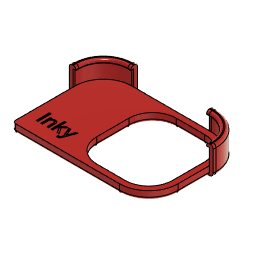
De-Anza-Merch-iPh-Case-Separate-Version v2 (Autodesk Fusion 360 design; units mm, degrees)
Autodesk Fusion 360 part; units mm, degrees
(part 1 of 2)
sketch "Body\\" plane through (0, 0, 0) normal (0, 0, 1) x (1, 0, 0)
  line L0 (0, 0) -> (72, 0)
  line L1 (0, 0) -> (0, 32)
  line L2 (0, 32) -> (-2, 32)
  line L3 (-2, 32) -> (-2, 33.5)
  line L4 (14.5, 50) -> (16, 50)
  line L5 (16, 50) -> (16, 48)
  line L6 (56, 48) -> (56, 50)
  line L7 (56, 50) -> (57.5, 50)
  line L8 (74, 33.5) -> (74, 32)
  line L9 (74, 32) -> (72, 32)
  line L10 (72, 32) -> (72, 0)
  line L11 (56.5, 3) -> (41.5, 3)
  line L12 (29, 15.5) -> (29, 32.5)
  line L13 (41.5, 45) -> (56.5, 45)
  line L14 (69, 32.5) -> (69, 15.5)
  line L15 (56, 48) -> (16, 48)
  arc A0 (14.5, 50) -> (-2, 33.5) centre (14.5, 33.5) ccw
  arc A1 (74, 33.5) -> (57.5, 50) centre (57.5, 33.5) ccw
  arc A2 (41.5, 45) -> (29, 32.5) centre (41.5, 32.5) ccw
  arc A3 (56.5, 3) -> (69, 15.5) centre (56.5, 15.5) ccw
  arc A4 (69, 32.5) -> (56.5, 45) centre (56.5, 32.5) ccw
  arc A5 (29, 15.5) -> (41.5, 3) centre (41.5, 15.5) ccw
  line L16 (32.6612, 41.3388) -> (65.3388, 6.6612) construction
  point P0 (74, 50)
  dimension "d2" = 72
  dimension "d3" = 40
  dimension "d5" = 42
  dimension "d6" = 3
  dimension "d15" = 48
  dimension "d16" = 3
  dimension "d27" = 16.5
  dimension "d28" = 16.5
  dimension "d29" = 12.5
  dimension "d30" = 12.5
  dimension "d31" = 2
  dimension "d32" = 2
  dimension "d33" = 2
  dimension "d34" = 2
  dimension "d35" = 12.5
  dimension "d36" = 12.5
  dimension "d38" = 18
  dimension "d39" = 18
  dimension "d40" = 18
  dimension "d41" = 18
  constraint perpendicular L1 L2
  constraint perpendicular L3 L4
  constraint perpendicular L4 L5
  constraint perpendicular L6 L7
  constraint perpendicular L7 L8
  constraint perpendicular L8 L9
  constraint perpendicular L0 L10
  constraint horizontal L11
  constraint vertical L12
  constraint horizontal L13
  constraint vertical L14
  constraint perpendicular L5 L15
  constraint coincident L0.start L1
  constraint coincident L5.end L15.end
  constraint coincident L0.start L1.start
  constraint coincident L1.start L0
  constraint tangent L4 A0
  constraint tangent L3 A0
  constraint coincident P0 L7
  constraint coincident P0 L8
  constraint tangent L7 A1
  constraint tangent L8 A1
  constraint tangent L13 A2
  constraint tangent L12 A2
  constraint tangent L11 A3
  constraint tangent L14 A3
  constraint vertical L6
  constraint tangent L13 A4
  constraint tangent L14 A4
  constraint tangent L11 A5
  constraint tangent L12 A5
  constraint midpoint A2 L16.start
  constraint midpoint A3 L16.end
  measures "d2" distance of L1 L10
  measures "d3" distance of L12 L14
  measures "d5" distance of L11 L13
  measures "d6" distance of L10 L14
  measures "d15" distance of L0 L15
  measures "d16" distance of L13 L15
  measures "d27" radius of A0
  measures "d28" radius of A1
  measures "d29" radius of A2
  measures "d30" radius of A3
  measures "d31" distance of L4 L15
  measures "d32" distance of L1 L3
  measures "d33" distance of L8 L10
  measures "d34" distance of L7 L15
  measures "d35" radius of A4
  measures "d36" radius of A5
  measures "d38" distance of L6 L8
  measures "d39" distance of L7 L9
  measures "d40" distance of L2 L4
  measures "d41" distance of L3 L5
extrude "Extrude1" add sketch "Body\\" along normal blind 4.5
sketch "Sketch5" plane through (0, 0, 4.5) normal (0, 0, 1) x (-1, 0, 0)
  arc A0 (-41.5, -45) -> (-29, -32.5) centre (-41.5, -32.5) ccw
  line L0 (-41.5, -45) -> (-56.5, -45)
  arc A1 (-69, -32.5) -> (-56.5, -45) centre (-56.5, -32.5) ccw
  line L1 (-69, -32.5) -> (-69, -15.5)
  arc A2 (-56.5, -3) -> (-69, -15.5) centre (-56.5, -15.5) ccw
  line L2 (-56.5, -3) -> (-41.5, -3)
  arc A3 (-29, -15.5) -> (-41.5, -3) centre (-41.5, -15.5) ccw
  line L3 (-29, -15.5) -> (-29, -32.5)
  line L4 (-74, -32) -> (-74, -33.5)
  arc A4 (-74, -33.5) -> (-57.5, -50) centre (-57.5, -33.5) ccw
  line L5 (-57.5, -50) -> (-56, -50)
  line L6 (-56, -50) -> (-56, -48)
  line L7 (-56, -48) -> (-16, -48)
  line L8 (-16, -48) -> (-16, -50)
  line L9 (-16, -50) -> (-14.5, -50)
  arc A5 (-14.5, -50) -> (2, -33.5) centre (-14.5, -33.5) ccw
  line L10 (2, -33.5) -> (2, -32)
  line L11 (2, -32) -> (0, -32)
  line L12 (0, -32) -> (0, 0)
  line L13 (0, 0) -> (-72, 0)
  line L14 (-72, 0) -> (-72, -32)
  line L15 (-72, -32) -> (-74, -32)
  line L16 (2, -32) -> (2, -33.5)
  line L17 (-14.5, -50) -> (-16, -50)
  line L18 (-16, -50) -> (-16, -46.5)
  line L19 (-1.5, -32) -> (-1.5, -33.5)
  line L20 (-14.5, -46.5) -> (-16, -46.5)
  line L21 (-1.5, -32) -> (2, -32)
  arc A6 (-14.5, -50) -> (2, -33.5) centre (-14.5, -33.5) ccw
  arc A7 (-14.5, -46.5) -> (-1.5, -33.5) centre (-14.5, -33.5) ccw
  line L22 (-36, -60) -> (-36, 25) construction
  line L23 (-56, -50) -> (-56, -46.5)
  arc A8 (-70.5, -33.5) -> (-57.5, -46.5) centre (-57.5, -33.5) ccw
  arc A9 (-74, -33.5) -> (-57.5, -50) centre (-57.5, -33.5) ccw
  line L24 (-57.5, -50) -> (-56, -50)
  line L25 (-57.5, -46.5) -> (-56, -46.5)
  line L26 (-70.5, -32) -> (-74, -32)
  line L27 (-74, -32) -> (-74, -33.5)
  line L28 (-70.5, -32) -> (-70.5, -33.5)
  dimension "d63" = 18
  dimension "d64" = 50
  dimension "d65" = 2
  dimension "d66" = 3.5
  dimension "d67" = 3.5
  dimension "d68" = 16.5
  dimension "d69" = 13
  dimension "d70" = 36
  constraint vertical L16
  constraint horizontal L17
  constraint vertical L18
  constraint vertical L19
  constraint horizontal L20
  constraint coincident L10.end L11.start
  constraint perpendicular L16 L21
  constraint tangent L16 A6
  constraint tangent L17 A6
  constraint tangent L19 A7
  constraint tangent L20 A7
  constraint vertical L22
  constraint symmetric L10.end L22 L4.start
  constraint symmetric L8.end L22 L5.end
  constraint symmetric L19.start L22 L26.start
  constraint symmetric L18.end L22 L23.end
  constraint symmetric A5.end L22 L4.end
  constraint symmetric L9.end L22 A4.end
  constraint symmetric A6 L22 A9
  constraint symmetric L19.end L22 A8.start
  constraint symmetric L20.start L22 A8.end
  constraint symmetric A7 L22 A8
  measures "d63" distance of L16 L18
  measures "d64" distance of L12.end L17
  measures "d65" distance of L12.end L16
  measures "d66" distance of L17 L20
  measures "d67" distance of L16 L19
  measures "d68" radius of A6
  measures "d69" radius of A7
  measures "d70" distance of L12.end L22
extrude "Extrude4" add sketch "Sketch5" along normal blind 10 contours L4 A4 L5 L6 L15 L23 A8 A9 L24 L25 L26 L27 L28 | L8 L9 A5 L10 L11 L16 L17 L18 L19 L20 L21 A6 A7
sketch "Sketch7" plane through (0, 0, 4.5) normal (0, 0, 1) x (-1, 0, 0)
  line L0 (-1.5, -32) -> (0, -32)
  line L1 (0, -32) -> (0, 0)
  line L2 (0, 0) -> (-72, 0)
  line L3 (-72, 0) -> (-72, -32)
  line L4 (-72, -32) -> (-70.5, -32)
  line L5 (-70.5, -32) -> (-70.5, -33.5)
  arc A0 (-70.5, -33.5) -> (-57.5, -46.5) centre (-57.5, -33.5) ccw
  line L6 (-57.5, -46.5) -> (-56, -46.5)
  line L7 (-56, -46.5) -> (-56, -48)
  line L8 (-56, -48) -> (-16, -48)
  line L9 (-16, -48) -> (-16, -46.5)
  line L10 (-16, -46.5) -> (-14.5, -46.5)
  arc A1 (-14.5, -46.5) -> (-1.5, -33.5) centre (-14.5, -33.5) ccw
  line L11 (-1.5, -33.5) -> (-1.5, -32)
  arc A2 (-41.5, -45) -> (-29, -32.5) centre (-41.5, -32.5) ccw
  line L12 (-41.5, -45) -> (-56.5, -45)
  arc A3 (-69, -32.5) -> (-56.5, -45) centre (-56.5, -32.5) ccw
  line L13 (-69, -32.5) -> (-69, -15.5)
  arc A4 (-56.5, -3) -> (-69, -15.5) centre (-56.5, -15.5) ccw
  line L14 (-56.5, -3) -> (-41.5, -3)
  arc A5 (-29, -15.5) -> (-41.5, -3) centre (-41.5, -15.5) ccw
  line L15 (-29, -15.5) -> (-29, -32.5)
  line L16 (0, -32) -> (-1.5, -32)
  line L17 (-16, -46.5) -> (-16, -48)
  line L18 (-16, -48) -> (-15, -48)
  line L19 (0, -33) -> (0, -32)
  line L20 (-1.5, -32) -> (-1.5, -33.5)
  line L21 (-14.5, -46.5) -> (-16, -46.5)
  arc A6 (-14.5, -46.5) -> (-1.5, -33.5) centre (-14.5, -33.5) ccw
  arc A7 (-15, -48) -> (0, -33) centre (-15, -33) ccw
  line L22 (-36, -60) -> (-36, 0) construction
  arc A8 (-70.5, -33.5) -> (-57.5, -46.5) centre (-57.5, -33.5) ccw
  line L23 (-70.5, -32) -> (-70.5, -33.5)
  arc A9 (-70.5, -33.5) -> (-57.5, -46.5) centre (-57.5, -33.5) ccw
  line L24 (-56, -46.5) -> (-56, -48)
  line L25 (-70.5, -32) -> (-72, -32)
  line L26 (-56, -48) -> (-57, -48)
  arc A10 (-72, -33) -> (-57, -48) centre (-57, -33) ccw
  line L27 (-72, -33) -> (-72, -32)
  line L28 (-57.5, -46.5) -> (-56, -46.5)
  line L29 (-72, -32) -> (-70.5, -32)
  line L30 (-56, -46.5) -> (-57.5, -46.5)
  line L31 (-56, -48) -> (-56, -46.5)
  line L32 (-70.5, -33.5) -> (-70.5, -32)
  dimension "d73" = 14.5
  dimension "d74" = 14.5
  dimension "d75" = 13
  dimension "d76" = 15
  dimension "d77" = 60
  dimension "d78" = 36
  constraint horizontal L16
  constraint vertical L17
  constraint horizontal L18
  constraint vertical L19
  constraint coincident L8.end L9.start
  constraint coincident L0.end L1.start
  constraint vertical L20
  constraint horizontal L21
  constraint tangent L20 A6
  constraint tangent L21 A6
  constraint tangent L18 A7
  constraint tangent L19 A7
  constraint vertical L22
  constraint coincident L2 L22.end
  constraint symmetric L0.start L22 L4.end
  constraint symmetric L0.end L22 L3.end
  constraint symmetric L8.end L22 L7.end
  constraint symmetric L9.end L22 L6.end
  constraint symmetric L10.end L22 A0.end
  constraint symmetric A1.end L22 L5.end
  constraint symmetric A1 L22 A9
  constraint symmetric A6 L22 A8
  constraint symmetric L18.end L22 L26.end
  constraint symmetric L19.start L22 A10.start
  constraint symmetric A7 L22 A10
  measures "d73" distance of L16 L21
  measures "d74" distance of L17 L20
  measures "d75" radius of A6
  measures "d76" radius of A7
  measures "d77" distance of L22.start L22.end
  measures "d78" distance of L1.end L22
extrude "Extrude5" cut sketch "Sketch7" along normal blind 8.3 contours L0 L9 L10 A1 L11 L16 L17 L18 L19 L20 L21 A6 A7 | L4 L5 A0 L6 L7 A8 L23 A9 L24 L25 L26 A10 L27 L28 L29 L30 L31 L32
fillet "Fillet1" radius 15.5 1 edges at (72, 0, 2.25)
fillet "Fillet2" radius 2 6 edges at (74, 32.75, 0) (69.1673, 45.1673, 0) (56.75, 50, 0) (15.25, 50, 0) (2.8327, 45.1673, 0) (-2, 32.75, 0)
fillet "Fillet3" radius 1.5 6 edges at (1.5, 32.75, 14.5) (5.3076, 42.6924, 14.5) (15.25, 46.5, 14.5) (56.75, 46.5, 14.5) (66.6924, 42.6924, 14.5) (70.5, 32.75, 14.5)
fillet "Fillet4" radius 1.5 6 edges at (15.25, 50, 14.5) (2.8327, 45.1673, 14.5) (-2, 32.75, 14.5) (74, 32.75, 14.5) (69.1673, 45.1673, 14.5) (56.75, 50, 14.5)
fillet "Fillet5" radius 1.5 8 edges at (69, 24, 0) (65.3388, 6.6612, 0) (49, 3, 0) (32.6612, 6.6612, 0) (29, 24, 0) (32.6612, 41.3388, 0) (49, 45, 0) (65.3388, 41.3388, 0)
fillet "Fillet6" radius 1.5 3 edges at (28.25, 0, 0) (67.4602, 4.5398, 0) (72, 23.75, 0)
fillet "Fillet7" radius 1.5 3 edges at (0, 0, 3) (0, 0.4393, 0.4393) (0, 16.75, 0)
sketch "Sketch8" plane through (0, 0, 0) normal (0, 0, -1) x (1, 0, 0)
  line L0 (1.5, -1.5) -> (1.5, -32)
  line L1 (1.5, -32) -> (0, -32)
  line L2 (0, -32) -> (0, -33.5)
  arc A0 (0, -33.5) -> (14.5, -48) centre (14.5, -33.5) ccw
  line L3 (14.5, -48) -> (16, -48)
  line L4 (16, -48) -> (56, -48)
  line L5 (56, -48) -> (57.5, -48)
  arc A1 (57.5, -48) -> (72, -33.5) centre (57.5, -33.5) ccw
  line L6 (72, -33.5) -> (72, -32)
  line L7 (72, -32) -> (70.5, -32)
  line L8 (70.5, -32) -> (70.5, -32.5)
  arc A2 (56.5, -46.5) -> (70.5, -32.5) centre (56.5, -32.5) ccw
  line L9 (56.5, -46.5) -> (41.5, -46.5)
  arc A3 (27.5, -32.5) -> (41.5, -46.5) centre (41.5, -32.5) ccw
  line L10 (27.5, -32.5) -> (27.5, -15.5)
  arc A4 (41.5, -1.5) -> (27.5, -15.5) centre (41.5, -15.5) ccw
  line L11 (41.5, -1.5) -> (1.5, -1.5)
  arc A5 (24.5, -32.5) -> (29.9783, -45) centre (41.5, -32.5) ccw
  line L12 (24.5, -32.5) -> (24.5, -15.5)
  arc A6 (28.5385, -4.5) -> (24.5, -15.5) centre (41.5, -15.5) ccw
  line L13 (28.5385, -4.5) -> (4.5, -4.5)
  line L14 (4.5, -4.5) -> (4.5, -35)
  line L15 (4.5, -35) -> (3.0982, -35)
  arc A7 (3.0982, -35) -> (14.5, -45) centre (14.5, -33.5) ccw
  line L16 (14.5, -45) -> (16, -45)
  line L17 (16, -45) -> (29.9783, -45)
  dimension "d95" = -3
extrude "Extrude6" cut sketch "Sketch8" against normal blind 1 contours A5 L12 A6 L13 L14 L15 A7 L16 L17
sketch "Sketch9" plane through (0, 0, 1) normal (0, 0, -1) x (1, 0, 0)
  line L0 (28.5385, -4.5) -> (4.5, -4.5)
  line L1 (4.5, -4.5) -> (4.5, -35)
  line L2 (4.5, -35) -> (3.0982, -35)
  arc A0 (3.0982, -35) -> (14.5, -45) centre (14.5, -33.5) ccw
  line L3 (14.5, -45) -> (29.9783, -45)
  arc A1 (24.5, -32.5) -> (29.9783, -45) centre (41.5, -32.5) ccw
  line L4 (24.5, -32.5) -> (24.5, -15.5)
  arc A2 (28.5385, -4.5) -> (24.5, -15.5) centre (41.5, -15.5) ccw
  spline S0 degree 3 poles (21.3936, -39.5443) (21.4725, -39.4567) (21.6302, -39.1939) (21.7353, -38.9574) knots 0 0 0 0 1 1 1 1
  spline S1 degree 3 poles (21.7353, -38.9574) (21.9018, -38.5894) (21.9368, -38.3704) (21.9368, -37.5994) knots 0 0 0 0 1 1 1 1
  spline S2 degree 3 poles (21.9368, -37.5994) (21.9368, -36.7233) (21.9193, -36.6532) (21.6477, -36.1538) knots 0 0 0 0 1 1 1 1
  spline S3 degree 3 poles (21.6477, -36.1538) (21.49, -35.8559) (21.1395, -35.3302) (20.8767, -34.971) knots 0 0 0 0 1 1 1 1
  spline S4 degree 3 poles (20.8767, -34.971) (20.4474, -34.4015) (20.4036, -34.3052) (20.4825, -34.1212) knots 0 0 0 0 1 1 1 1
  spline S5 degree 3 poles (20.4825, -34.1212) (20.6139, -33.8321) (20.6051, -33.0961) (20.4474, -32.3076) knots 0 0 0 0 1 1 1 1
  spline S6 degree 3 poles (20.4474, -32.3076) (20.2459, -31.2125) (19.7903, -30.3802) (19.2647, -30.1086) knots 0 0 0 0 1 1 1 1
  spline S7 degree 3 poles (19.2647, -30.1086) (19.1157, -30.0297) (18.923, -29.8195) (18.8354, -29.6355) knots 0 0 0 0 1 1 1 1
  spline S8 degree 3 poles (18.8354, -29.6355) (18.739, -29.4515) (18.4499, -29.1098) (18.1958, -28.8732) knots 0 0 0 0 1 1 1 1
  spline S9 degree 3 poles (18.1958, -28.8732) (17.7753, -28.4965) (17.6876, -28.3476) (17.4336, -27.6116) knots 0 0 0 0 1 1 1 1
  spline S10 degree 3 poles (17.4336, -27.6116) (17.0831, -26.6216) (16.6451, -25.728) (16.3297, -25.3513) knots 0 0 0 0 1 1 1 1
  spline S11 degree 3 poles (16.3297, -25.3513) (15.9792, -24.9307) (15.62, -24.8519) (14.1394, -24.8519) knots 0 0 0 0 1 1 1 1
  spline S12 degree 3 poles (14.1394, -24.8519) (12.65, -24.8606) (12.3433, -24.9395) (11.9578, -25.4389) knots 0 0 0 0 1 1 1 1
  spline S13 degree 3 poles (11.9578, -25.4389) (11.6775, -25.8068) (11.2219, -26.8056) (10.8977, -27.7431) knots 0 0 0 0 1 1 1 1
  spline S14 degree 3 poles (10.8977, -27.7431) (10.6962, -28.3301) (10.5823, -28.5053) (10.2319, -28.8207) knots 0 0 0 0 1 1 1 1
  spline S15 degree 3 poles (10.2319, -28.8207) (9.9953, -29.0309) (9.6975, -29.3814) (9.5748, -29.5917) knots 0 0 0 0 1 1 1 1
  spline S16 degree 3 poles (9.5748, -29.5917) (9.4434, -29.8107) (9.2331, -30.0385) (9.0929, -30.1086) knots 0 0 0 0 1 1 1 1
  spline S17 degree 3 poles (9.0929, -30.1086) (8.576, -30.3802) (8.1204, -31.2212) (7.9189, -32.3076) knots 0 0 0 0 1 1 1 1
  spline S18 degree 3 poles (7.9189, -32.3076) (7.7612, -33.0961) (7.7525, -33.7007) (7.8839, -34.0686) knots 0 0 0 0 1 1 1 1
  spline S19 degree 3 poles (7.8839, -34.0686) (7.9627, -34.3139) (7.9365, -34.384) (7.4896, -34.9798) knots 0 0 0 0 1 1 1 1
  spline S20 degree 3 poles (7.4896, -34.9798) (6.7099, -36.0048) (6.4558, -36.5656) (6.4033, -37.2927) knots 0 0 0 0 1 1 1 1
  spline S21 degree 3 poles (6.4033, -37.2927) (6.3595, -38.0024) (6.5259, -38.7033) (6.8501, -39.1851) knots 0 0 0 0 1 1 1 1
  spline S22 degree 3 poles (6.8501, -39.1851) (7.0253, -39.4567) (7.0954, -39.483) (7.5159, -39.5093) knots 0 0 0 0 1 1 1 1
  spline S23 degree 3 poles (7.5159, -39.5093) (8.0854, -39.5443) (8.6987, -39.3516) (9.2857, -38.9486) knots 0 0 0 0 1 1 1 1
  spline S24 degree 3 poles (9.2857, -38.9486) (9.6098, -38.7383) (9.7675, -38.677) (9.8727, -38.7296) knots 0 0 0 0 1 1 1 1
  spline S25 degree 3 poles (9.8727, -38.7296) (9.9603, -38.7734) (10.337, -38.896) (10.7225, -39.0099) knots 0 0 0 0 1 1 1 1
  spline S26 degree 3 poles (10.7225, -39.0099) (11.6775, -39.2815) (13.4648, -39.3078) (13.8853, -39.0537) knots 0 0 0 0 1 1 1 1
  spline S27 degree 3 poles (13.8853, -39.0537) (14.1569, -38.896) (14.1744, -38.896) (14.5424, -39.045) knots 0 0 0 0 1 1 1 1
  spline S28 degree 3 poles (14.5424, -39.045) (15.3747, -39.3779) (16.8378, -39.2903) (18.2046, -38.8259) knots 0 0 0 0 1 1 1 1
  line L5 (18.2046, -38.8259) -> (18.6864, -38.6682)
  line L6 (18.6864, -38.6682) -> (18.9931, -38.9135)
  spline S29 degree 3 poles (18.9931, -38.9135) (19.8779, -39.6144) (21.0519, -39.9211) (21.3936, -39.5443) knots 0 0 0 0 1 1 1 1
  spline S30 degree 3 poles (20.1671, -38.8172) (19.9655, -38.7208) (19.5976, -38.458) (19.361, -38.2477) knots 0 0 0 0 1 1 1 1
  spline S31 degree 3 poles (19.361, -38.2477) (18.9405, -37.8622) (18.9142, -37.8534) (18.6777, -37.9761) knots 0 0 0 0 1 1 1 1
  spline S32 degree 3 poles (18.6777, -37.9761) (18.5462, -38.0462) (18.0731, -38.2302) (17.6438, -38.3879) knots 0 0 0 0 1 1 1 1
  spline S33 degree 3 poles (17.6438, -38.3879) (16.9692, -38.6332) (16.6976, -38.677) (15.7865, -38.712) knots 0 0 0 0 1 1 1 1
  spline S34 degree 3 poles (15.7865, -38.712) (14.7527, -38.7646) (14.7176, -38.7558) (14.5073, -38.5456) knots 0 0 0 0 1 1 1 1
  spline S35 degree 3 poles (14.5073, -38.5456) (14.3934, -38.4317) (14.2708, -38.274) (14.2357, -38.2039) knots 0 0 0 0 1 1 1 1
  spline S36 degree 3 poles (14.2357, -38.2039) (14.1919, -38.0988) (14.1744, -38.0988) (14.1306, -38.2039) knots 0 0 0 0 1 1 1 1
  spline S37 degree 3 poles (14.1306, -38.2039) (14.0956, -38.274) (13.9729, -38.4317) (13.859, -38.5456) knots 0 0 0 0 1 1 1 1
  spline S38 degree 3 poles (13.859, -38.5456) (13.6487, -38.7558) (13.6137, -38.7558) (12.6237, -38.7208) knots 0 0 0 0 1 1 1 1
  spline S39 degree 3 poles (12.6237, -38.7208) (11.7651, -38.6858) (11.4585, -38.6332) (10.7576, -38.3966) knots 0 0 0 0 1 1 1 1
  spline S40 degree 3 poles (10.7576, -38.3966) (10.2932, -38.2389) (9.8026, -38.0374) (9.6624, -37.9586) knots 0 0 0 0 1 1 1 1
  line L7 (9.6624, -37.9586) -> (9.4083, -37.8009)
  line L8 (9.4083, -37.8009) -> (8.8827, -38.2915)
  spline S41 degree 3 poles (8.8827, -38.2915) (8.3044, -38.8259) (7.7087, -39.0975) (7.4546, -38.9486) knots 0 0 0 0 1 1 1 1
  spline S42 degree 3 poles (7.4546, -38.9486) (7.148, -38.7646) (6.9114, -38.125) (6.9114, -37.4592) knots 0 0 0 0 1 1 1 1
  spline S43 degree 3 poles (6.9114, -37.4592) (6.9114, -36.8897) (6.9377, -36.7933) (7.2443, -36.3202) knots 0 0 0 0 1 1 1 1
  spline S44 degree 3 poles (7.2443, -36.3202) (7.4371, -36.0311) (7.8226, -35.523) (8.1117, -35.19) knots 0 0 0 0 1 1 1 1
  spline S45 degree 3 poles (8.1117, -35.19) (8.7863, -34.3928) (8.7775, -34.4103) (8.6111, -34.0861) knots 0 0 0 0 1 1 1 1
  spline S46 degree 3 poles (8.6111, -34.0861) (8.4008, -33.6656) (8.4797, -32.5442) (8.7775, -31.8871) knots 0 0 0 0 1 1 1 1
  spline S47 degree 3 poles (8.7775, -31.8871) (8.9878, -31.414) (9.6449, -30.5904) (9.8114, -30.5904) knots 0 0 0 0 1 1 1 1
  spline S48 degree 3 poles (9.8114, -30.5904) (9.8552, -30.5904) (9.8902, -30.7394) (9.8902, -30.9234) knots 0 0 0 0 1 1 1 1
  spline S49 degree 3 poles (9.8902, -30.9234) (9.8902, -31.3264) (10.1443, -31.8783) (10.4422, -32.1587) knots 0 0 0 0 1 1 1 1
  spline S50 degree 3 poles (10.4422, -32.1587) (10.6524, -32.3514) (10.7225, -32.3602) (11.3095, -32.3164) knots 0 0 0 0 1 1 1 1
  spline S51 degree 3 poles (11.3095, -32.3164) (11.66, -32.2901) (12.0192, -32.2463) (12.098, -32.2113) knots 0 0 0 0 1 1 1 1
  spline S52 degree 3 poles (12.098, -32.2113) (12.2382, -32.1587) (12.2557, -32.2025) (12.2557, -32.5705) knots 0 0 0 0 1 1 1 1
  spline S53 degree 3 poles (12.2557, -32.5705) (12.2557, -32.807) (12.3346, -33.3152) (12.4222, -33.7007) knots 0 0 0 0 1 1 1 1
  spline S54 degree 3 poles (12.4222, -33.7007) (12.5186, -34.0861) (12.5799, -34.4103) (12.5624, -34.4278) knots 0 0 0 0 1 1 1 1
  spline S55 degree 3 poles (12.5624, -34.4278) (12.5448, -34.4453) (12.4572, -34.4191) (12.3609, -34.3665) knots 0 0 0 0 1 1 1 1
  spline S56 degree 3 poles (12.3609, -34.3665) (12.1068, -34.2351) (11.4672, -34.2526) (11.2044, -34.4015) knots 0 0 0 0 1 1 1 1
  spline S57 degree 3 poles (11.2044, -34.4015) (10.9415, -34.5505) (10.4772, -34.568) (10.2144, -34.4366) knots 0 0 0 0 1 1 1 1
  spline S58 degree 3 poles (10.2144, -34.4366) (10.0304, -34.3402) (10.0304, -34.349) (10.2319, -34.568) knots 0 0 0 0 1 1 1 1
  spline S59 degree 3 poles (10.2319, -34.568) (10.3545, -34.6907) (10.5035, -34.7958) (10.5736, -34.7958) knots 0 0 0 0 1 1 1 1
  spline S60 degree 3 poles (10.5736, -34.7958) (10.6612, -34.7958) (10.6787, -34.8484) (10.6349, -34.9535) knots 0 0 0 0 1 1 1 1
  spline S61 degree 3 poles (10.6349, -34.9535) (10.5999, -35.0323) (10.5122, -35.2777) (10.4509, -35.4879) knots 0 0 0 0 1 1 1 1
  spline S62 degree 3 poles (10.4509, -35.4879) (10.3808, -35.707) (10.2669, -35.9786) (10.1881, -36.0924) knots 0 0 0 0 1 1 1 1
  spline S63 degree 3 poles (10.1881, -36.0924) (9.9866, -36.3991) (10.0829, -36.4166) (10.5561, -36.1275) knots 0 0 0 0 1 1 1 1
  spline S64 degree 3 poles (10.5561, -36.1275) (10.8627, -35.9435) (11.143, -35.8559) (11.5198, -35.8209) knots 0 0 0 0 1 1 1 1
  spline S65 degree 3 poles (11.5198, -35.8209) (11.8089, -35.7946) (12.1769, -35.7157) (12.3258, -35.6369) knots 0 0 0 0 1 1 1 1
  line L9 (12.3258, -35.6369) -> (12.6062, -35.4879)
  line L10 (12.6062, -35.4879) -> (12.6149, -35.7332)
  spline S66 degree 3 poles (12.6149, -35.7332) (12.6149, -35.9698) (12.6237, -35.961) (12.7814, -35.6281) knots 0 0 0 0 1 1 1 1
  spline S67 degree 3 poles (12.7814, -35.6281) (12.9917, -35.1725) (12.9917, -34.6381) (12.7814, -33.8321) knots 0 0 0 0 1 1 1 1
  spline S68 degree 3 poles (12.7814, -33.8321) (12.5273, -32.8508) (12.501, -32.8946) (13.2808, -32.8333) knots 0 0 0 0 1 1 1 1
  spline S69 degree 3 poles (13.2808, -32.8333) (14.1306, -32.7632) (14.2357, -32.7632) (15.0768, -32.8333) knots 0 0 0 0 1 1 1 1
  spline S70 degree 3 poles (15.0768, -32.8333) (15.8741, -32.8946) (15.8478, -32.8508) (15.585, -33.8846) knots 0 0 0 0 1 1 1 1
  spline S71 degree 3 poles (15.585, -33.8846) (15.3747, -34.7345) (15.3659, -34.9973) (15.5587, -35.5493) knots 0 0 0 0 1 1 1 1
  spline S72 degree 3 poles (15.5587, -35.5493) (15.6989, -35.9347) (15.7164, -35.9523) (15.7427, -35.742) knots 0 0 0 0 1 1 1 1
  spline S73 degree 3 poles (15.7427, -35.742) (15.7602, -35.6018) (15.7777, -35.4967) (15.7952, -35.4967) knots 0 0 0 0 1 1 1 1
  spline S74 degree 3 poles (15.7952, -35.4967) (15.804, -35.4967) (15.9617, -35.5755) (16.1544, -35.6719) knots 0 0 0 0 1 1 1 1
  spline S75 degree 3 poles (16.1544, -35.6719) (16.3647, -35.777) (16.6713, -35.8471) (16.9605, -35.8471) knots 0 0 0 0 1 1 1 1
  spline S76 degree 3 poles (16.9605, -35.8471) (17.3284, -35.8471) (17.4949, -35.8997) (17.8191, -36.1187) knots 0 0 0 0 1 1 1 1
  spline S77 degree 3 poles (17.8191, -36.1187) (18.0381, -36.2677) (18.2396, -36.3728) (18.2659, -36.3465) knots 0 0 0 0 1 1 1 1
  spline S78 degree 3 poles (18.2659, -36.3465) (18.2834, -36.329) (18.2396, -36.1888) (18.152, -36.0311) knots 0 0 0 0 1 1 1 1
  spline S79 degree 3 poles (18.152, -36.0311) (18.0381, -35.8384) (17.933, -35.7595) (17.7665, -35.7595) knots 0 0 0 0 1 1 1 1
  spline S80 degree 3 poles (17.7665, -35.7595) (17.5124, -35.7595) (17.3372, -35.6106) (17.3372, -35.4003) knots 0 0 0 0 1 1 1 1
  spline S81 degree 3 poles (17.3372, -35.4003) (17.3372, -34.9447) (16.61, -34.5768) (16.1282, -34.787) knots 0 0 0 0 1 1 1 1
  line L11 (16.1282, -34.787) -> (15.8916, -34.8834)
  line L12 (15.8916, -34.8834) -> (16.1019, -34.7082)
  spline S82 degree 3 poles (16.1019, -34.7082) (16.2333, -34.5943) (16.4348, -34.533) (16.6538, -34.533) knots 0 0 0 0 1 1 1 1
  spline S83 degree 3 poles (16.6538, -34.533) (17.013, -34.533) (17.346, -34.7783) (17.7052, -35.3215) knots 0 0 0 0 1 1 1 1
  spline S84 degree 3 poles (17.7052, -35.3215) (17.8366, -35.523) (17.8541, -35.523) (17.8541, -35.3653) knots 0 0 0 0 1 1 1 1
  spline S85 degree 3 poles (17.8541, -35.3653) (17.8629, -35.2689) (17.8278, -35.1287) (17.7753, -35.0586) knots 0 0 0 0 1 1 1 1
  spline S86 degree 3 poles (17.7753, -35.0586) (17.7227, -34.9623) (17.7665, -34.8746) (17.9768, -34.6994) knots 0 0 0 0 1 1 1 1
  line L13 (17.9768, -34.6994) -> (18.2571, -34.4629)
  line L14 (18.2571, -34.4629) -> (17.8541, -34.5067)
  spline S87 degree 3 poles (17.8541, -34.5067) (17.5825, -34.5417) (17.3635, -34.5067) (17.1795, -34.4103) knots 0 0 0 0 1 1 1 1
  spline S88 degree 3 poles (17.1795, -34.4103) (16.8641, -34.2526) (16.2683, -34.2263) (16.0055, -34.3665) knots 0 0 0 0 1 1 1 1
  spline S89 degree 3 poles (16.0055, -34.3665) (15.9091, -34.4191) (15.8215, -34.4453) (15.804, -34.4278) knots 0 0 0 0 1 1 1 1
  spline S90 degree 3 poles (15.804, -34.4278) (15.7865, -34.4103) (15.8478, -34.0861) (15.9354, -33.7007) knots 0 0 0 0 1 1 1 1
  spline S91 degree 3 poles (15.9354, -33.7007) (16.0318, -33.3152) (16.1019, -32.807) (16.1106, -32.5705) knots 0 0 0 0 1 1 1 1
  spline S92 degree 3 poles (16.1106, -32.5705) (16.1106, -32.2025) (16.1282, -32.1587) (16.2596, -32.2113) knots 0 0 0 0 1 1 1 1
  spline S93 degree 3 poles (16.2596, -32.2113) (16.3472, -32.2463) (16.7064, -32.2989) (17.0568, -32.3251) knots 0 0 0 0 1 1 1 1
  spline S94 degree 3 poles (17.0568, -32.3251) (17.6701, -32.3602) (17.7052, -32.3602) (17.968, -32.1149) knots 0 0 0 0 1 1 1 1
  spline S95 degree 3 poles (17.968, -32.1149) (18.3009, -31.7995) (18.4761, -31.3965) (18.4761, -30.9409) knots 0 0 0 0 1 1 1 1
  spline S96 degree 3 poles (18.4761, -30.9409) (18.4761, -30.7481) (18.5112, -30.5904) (18.555, -30.5904) knots 0 0 0 0 1 1 1 1
  spline S97 degree 3 poles (18.555, -30.5904) (18.7127, -30.5904) (19.3785, -31.414) (19.5976, -31.8871) knots 0 0 0 0 1 1 1 1
  spline S98 degree 3 poles (19.5976, -31.8871) (19.8867, -32.5354) (19.9743, -33.6568) (19.7553, -34.0774) knots 0 0 0 0 1 1 1 1
  spline S99 degree 3 poles (19.7553, -34.0774) (19.6764, -34.2263) (19.6151, -34.3665) (19.6151, -34.3928) knots 0 0 0 0 1 1 1 1
  spline S100 degree 3 poles (19.6151, -34.3928) (19.6151, -34.4103) (19.9042, -34.7695) (20.2459, -35.1725) knots 0 0 0 0 1 1 1 1
  spline S101 degree 3 poles (20.2459, -35.1725) (21.1133, -36.1801) (21.5426, -36.916) (21.5426, -37.3979) knots 0 0 0 0 1 1 1 1
  spline S102 degree 3 poles (21.5426, -37.3979) (21.5426, -37.8622) (21.3148, -38.5456) (21.0782, -38.8084) knots 0 0 0 0 1 1 1 1
  spline S103 degree 3 poles (21.0782, -38.8084) (20.8592, -39.045) (20.6489, -39.0537) (20.1671, -38.8172) knots 0 0 0 0 1 1 1 1
  spline S104 degree 3 poles (10.7576, -35.2514) (11.0116, -34.752) (11.327, -34.533) (11.7739, -34.533) knots 0 0 0 0 1 1 1 1
  spline S105 degree 3 poles (11.7739, -34.533) (12.0367, -34.533) (12.1856, -34.5855) (12.3083, -34.7169) knots 0 0 0 0 1 1 1 1
  spline S106 degree 3 poles (12.3083, -34.7169) (12.4747, -34.9009) (12.4747, -34.9009) (12.2382, -34.7958) knots 0 0 0 0 1 1 1 1
  spline S107 degree 3 poles (12.2382, -34.7958) (11.7476, -34.568) (11.0292, -34.9447) (11.0292, -35.4266) knots 0 0 0 0 1 1 1 1
  spline S108 degree 3 poles (11.0292, -35.4266) (11.0292, -35.5931) (10.6612, -35.8033) (10.6086, -35.6719) knots 0 0 0 0 1 1 1 1
  spline S109 degree 3 poles (10.6086, -35.6719) (10.5911, -35.6281) (10.6612, -35.4441) (10.7576, -35.2514) knots 0 0 0 0 1 1 1 1
  spline S110 degree 3 poles (16.5837, -35.19) (16.5925, -34.8308) (16.6626, -34.8046) (16.8466, -35.0762) knots 0 0 0 0 1 1 1 1
  spline S111 degree 3 poles (16.8466, -35.0762) (17.0393, -35.3565) (17.0218, -35.4967) (16.7852, -35.4967) knots 0 0 0 0 1 1 1 1
  spline S112 degree 3 poles (16.7852, -35.4967) (16.61, -35.4967) (16.5837, -35.4529) (16.5837, -35.19) knots 0 0 0 0 1 1 1 1
  spline S113 degree 3 poles (11.3796, -35.3828) (11.3796, -35.2514) (11.6249, -34.8834) (11.7125, -34.8834) knots 0 0 0 0 1 1 1 1
  spline S114 degree 3 poles (11.7125, -34.8834) (11.7476, -34.8834) (11.7739, -35.0236) (11.7826, -35.19) knots 0 0 0 0 1 1 1 1
  spline S115 degree 3 poles (11.7826, -35.19) (11.7826, -35.4529) (11.7563, -35.4967) (11.5811, -35.4967) knots 0 0 0 0 1 1 1 1
  spline S116 degree 3 poles (11.5811, -35.4967) (11.4672, -35.4967) (11.3796, -35.4441) (11.3796, -35.3828) knots 0 0 0 0 1 1 1 1
  spline S117 degree 3 poles (16.0843, -31.8696) (15.7339, -31.7557) (15.2608, -31.6418) (15.033, -31.6067) knots 0 0 0 0 1 1 1 1
  spline S118 degree 3 poles (15.033, -31.6067) (14.3496, -31.5191) (14.2708, -31.449) (14.2708, -30.8971) knots 0 0 0 0 1 1 1 1
  spline S119 degree 3 poles (14.2708, -30.8971) (14.2708, -30.4327) (14.2795, -30.4152) (14.5073, -30.4152) knots 0 0 0 0 1 1 1 1
  spline S120 degree 3 poles (14.5073, -30.4152) (15.0505, -30.4152) (15.8303, -30.091) (16.5487, -29.5741) knots 0 0 0 0 1 1 1 1
  spline S121 degree 3 poles (16.5487, -29.5741) (17.0218, -29.2412) (17.1444, -29.2149) (17.5299, -29.4164) knots 0 0 0 0 1 1 1 1
  line L15 (17.5299, -29.4164) -> (17.8103, -29.5654)
  line L16 (17.8103, -29.5654) -> (17.2496, -29.8107)
  spline S122 degree 3 poles (17.2496, -29.8107) (16.9429, -29.9509) (16.7152, -30.091) (16.7502, -30.1173) knots 0 0 0 0 1 1 1 1
  spline S123 degree 3 poles (16.7502, -30.1173) (16.7765, -30.1436) (17.0043, -30.1173) (17.2671, -30.0648) knots 0 0 0 0 1 1 1 1
  spline S124 degree 3 poles (17.2671, -30.0648) (17.8716, -29.9246) (18.1607, -29.9684) (18.1958, -30.1962) knots 0 0 0 0 1 1 1 1
  spline S125 degree 3 poles (18.1958, -30.1962) (18.2133, -30.3539) (18.1432, -30.3889) (17.5387, -30.4853) knots 0 0 0 0 1 1 1 1
  spline S126 degree 3 poles (17.5387, -30.4853) (16.5662, -30.6342) (16.5224, -30.7657) (17.4511, -30.7657) knots 0 0 0 0 1 1 1 1
  line L17 (17.4511, -30.7657) -> (18.2133, -30.7657)
  line L18 (18.2133, -30.7657) -> (18.2133, -31.0197)
  spline S127 degree 3 poles (18.2133, -31.0197) (18.2133, -31.3176) (18.0293, -31.3789) (16.9955, -31.3877) knots 0 0 0 0 1 1 1 1
  spline S128 degree 3 poles (16.9955, -31.3877) (16.1106, -31.3965) (16.4348, -31.5366) (17.3547, -31.5454) knots 0 0 0 0 1 1 1 1
  spline S129 degree 3 poles (17.3547, -31.5454) (17.7314, -31.5542) (18.0381, -31.5804) (18.0381, -31.6155) knots 0 0 0 0 1 1 1 1
  spline S130 degree 3 poles (18.0381, -31.6155) (18.0381, -31.6505) (17.9505, -31.7644) (17.8453, -31.8783) knots 0 0 0 0 1 1 1 1
  spline S131 degree 3 poles (17.8453, -31.8783) (17.5913, -32.1499) (16.9254, -32.1499) (16.0843, -31.8696) knots 0 0 0 0 1 1 1 1
  spline S132 degree 3 poles (10.5298, -31.8871) (10.4159, -31.782) (10.3283, -31.6681) (10.3283, -31.6243) knots 0 0 0 0 1 1 1 1
  spline S133 degree 3 poles (10.3283, -31.6243) (10.3283, -31.5892) (10.6349, -31.5542) (11.0029, -31.5454) knots 0 0 0 0 1 1 1 1
  spline S134 degree 3 poles (11.0029, -31.5454) (11.9666, -31.5366) (12.2382, -31.3965) (11.3358, -31.3789) knots 0 0 0 0 1 1 1 1
  spline S135 degree 3 poles (11.3358, -31.3789) (10.3896, -31.3527) (10.2056, -31.3001) (10.1706, -31.0022) knots 0 0 0 0 1 1 1 1
  line L19 (10.1706, -31.0022) -> (10.1443, -30.7657)
  line L20 (10.1443, -30.7657) -> (10.9065, -30.7657)
  spline S136 degree 3 poles (10.9065, -30.7657) (11.8439, -30.7657) (11.8001, -30.643) (10.8276, -30.4853) knots 0 0 0 0 1 1 1 1
  spline S137 degree 3 poles (10.8276, -30.4853) (10.1706, -30.3889) (10.0742, -30.3188) (10.2319, -30.0735) knots 0 0 0 0 1 1 1 1
  spline S138 degree 3 poles (10.2319, -30.0735) (10.3283, -29.9246) (10.9503, -29.9772) (11.5811, -30.1962) knots 0 0 0 0 1 1 1 1
  spline S139 degree 3 poles (11.5811, -30.1962) (12.0192, -30.3451) (12.282, -30.3101) (11.8965, -30.1611) knots 0 0 0 0 1 1 1 1
  spline S140 degree 3 poles (11.8965, -30.1611) (11.7826, -30.1173) (11.4322, -29.9596) (11.1255, -29.8195) knots 0 0 0 0 1 1 1 1
  line L21 (11.1255, -29.8195) -> (10.5561, -29.5654)
  line L22 (10.5561, -29.5654) -> (10.8364, -29.4164)
  spline S141 degree 3 poles (10.8364, -29.4164) (11.2219, -29.2149) (11.3446, -29.2412) (11.8177, -29.5741) knots 0 0 0 0 1 1 1 1
  spline S142 degree 3 poles (11.8177, -29.5741) (12.5361, -30.091) (13.3158, -30.4152) (13.8503, -30.4152) knots 0 0 0 0 1 1 1 1
  spline S143 degree 3 poles (13.8503, -30.4152) (14.0868, -30.4152) (14.0956, -30.4327) (14.0956, -30.9058) knots 0 0 0 0 1 1 1 1
  spline S144 degree 3 poles (14.0956, -30.9058) (14.0956, -31.3702) (14.0868, -31.3877) (13.7889, -31.5191) knots 0 0 0 0 1 1 1 1
  spline S145 degree 3 poles (13.7889, -31.5191) (13.6225, -31.5804) (13.3596, -31.6418) (13.2019, -31.6418) knots 0 0 0 0 1 1 1 1
  spline S146 degree 3 poles (13.2019, -31.6418) (13.0442, -31.6505) (12.6324, -31.7469) (12.2995, -31.8608) knots 0 0 0 0 1 1 1 1
  spline S147 degree 3 poles (12.2995, -31.8608) (11.4935, -32.1412) (10.8101, -32.1499) (10.5298, -31.8871) knots 0 0 0 0 1 1 1 1
  line L23 (15.3221, -29.1273) -> (15.3309, -28.4439)
  line L24 (15.3309, -28.4439) -> (15.4973, -28.6455)
  spline S148 degree 3 poles (15.4973, -28.6455) (15.7602, -28.9609) (15.9004, -29.5041) (15.7602, -29.6705) knots 0 0 0 0 1 1 1 1
  spline S149 degree 3 poles (15.7602, -29.6705) (15.6989, -29.7406) (15.5762, -29.8019) (15.4886, -29.8019) knots 0 0 0 0 1 1 1 1
  spline S150 degree 3 poles (15.4886, -29.8019) (15.3396, -29.8019) (15.3221, -29.7318) (15.3221, -29.1273) knots 0 0 0 0 1 1 1 1
  spline S151 degree 3 poles (12.6062, -29.6705) (12.5098, -29.5566) (12.5186, -29.469) (12.6149, -29.1711) knots 0 0 0 0 1 1 1 1
  spline S152 degree 3 poles (12.6149, -29.1711) (12.6763, -28.9784) (12.7989, -28.7331) (12.8865, -28.6279) knots 0 0 0 0 1 1 1 1
  spline S153 degree 3 poles (12.8865, -28.6279) (13.0355, -28.4527) (13.0355, -28.4615) (13.0442, -29.1273) knots 0 0 0 0 1 1 1 1
  spline S154 degree 3 poles (13.0442, -29.1273) (13.0442, -29.7318) (13.0267, -29.8019) (12.8778, -29.8019) knots 0 0 0 0 1 1 1 1
  spline S155 degree 3 poles (12.8778, -29.8019) (12.7901, -29.8019) (12.6675, -29.7406) (12.6062, -29.6705) knots 0 0 0 0 1 1 1 1
  spline S156 degree 3 poles (16.829, -28.6455) (16.7852, -28.5841) (16.4786, -28.0234) (16.1544, -27.4101) knots 0 0 0 0 1 1 1 1
  line L25 (16.1544, -27.4101) -> (15.5587, -26.2799)
  line L26 (15.5587, -26.2799) -> (15.1995, -26.3413)
  spline S157 degree 3 poles (15.1995, -26.3413) (14.7176, -26.4201) (13.5962, -26.4201) (13.237, -26.3413) knots 0 0 0 0 1 1 1 1
  spline S158 degree 3 poles (13.237, -26.3413) (12.8515, -26.2537) (12.7726, -26.3413) (12.2557, -27.34) knots 0 0 0 0 1 1 1 1
  spline S159 degree 3 poles (12.2557, -27.34) (11.7038, -28.4177) (11.4935, -28.7506) (11.3796, -28.7506) knots 0 0 0 0 1 1 1 1
  spline S160 degree 3 poles (11.3796, -28.7506) (11.2394, -28.7506) (11.2745, -28.4702) (11.5198, -27.7343) knots 0 0 0 0 1 1 1 1
  spline S161 degree 3 poles (11.5198, -27.7343) (11.8702, -26.683) (12.2908, -25.8244) (12.5624, -25.6141) knots 0 0 0 0 1 1 1 1
  spline S162 degree 3 poles (12.5624, -25.6141) (12.7901, -25.4301) (12.8953, -25.4213) (14.1919, -25.4213) knots 0 0 0 0 1 1 1 1
  spline S163 degree 3 poles (14.1919, -25.4213) (15.5587, -25.4213) (15.5762, -25.4213) (15.8478, -25.6579) knots 0 0 0 0 1 1 1 1
  spline S164 degree 3 poles (15.8478, -25.6579) (15.9967, -25.7806) (16.2245, -26.1047) (16.3472, -26.3763) knots 0 0 0 0 1 1 1 1
  spline S165 degree 3 poles (16.3472, -26.3763) (16.6451, -27.0422) (17.0744, -28.3388) (17.0744, -28.5666) knots 0 0 0 0 1 1 1 1
  spline S166 degree 3 poles (17.0744, -28.5666) (17.0744, -28.7769) (16.9692, -28.8032) (16.829, -28.6455) knots 0 0 0 0 1 1 1 1
  spline S167 degree 3 poles (14.9717, -27.121) (14.7527, -26.6216) (14.7527, -26.6304) (14.9892, -26.6654) knots 0 0 0 0 1 1 1 1
  spline S168 degree 3 poles (14.9892, -26.6654) (15.1644, -26.6917) (15.1907, -26.753) (15.217, -27.1123) knots 0 0 0 0 1 1 1 1
  spline S169 degree 3 poles (15.217, -27.1123) (15.2345, -27.34) (15.2258, -27.524) (15.1995, -27.524) knots 0 0 0 0 1 1 1 1
  spline S170 degree 3 poles (15.1995, -27.524) (15.1732, -27.524) (15.0768, -27.34) (14.9717, -27.121) knots 0 0 0 0 1 1 1 1
  spline S171 degree 3 poles (13.1669, -26.7706) (13.2107, -26.6654) (13.5699, -26.5866) (13.5699, -26.683) knots 0 0 0 0 1 1 1 1
  spline S172 degree 3 poles (13.5699, -26.683) (13.5699, -26.7005) (13.4823, -26.902) (13.3684, -27.1385) knots 0 0 0 0 1 1 1 1
  line L27 (13.3684, -27.1385) -> (13.1756, -27.5678)
  line L28 (13.1756, -27.5678) -> (13.1494, -27.2261)
  spline S173 degree 3 poles (13.1494, -27.2261) (13.1318, -27.0422) (13.1406, -26.8407) (13.1669, -26.7706) knots 0 0 0 0 1 1 1 1
  spline S174 degree 3 poles (20.8329, -38.2477) (21.1921, -37.7921) (20.9468, -36.7495) (20.3248, -36.0224) knots 0 0 0 0 1 1 1 1
  line L29 (20.3248, -36.0224) -> (20.132, -35.8033)
  line L30 (20.132, -35.8033) -> (20.2021, -36.11)
  spline S175 degree 3 poles (20.2021, -36.11) (20.2371, -36.2764) (20.2722, -36.6356) (20.2722, -36.8985) knots 0 0 0 0 1 1 1 1
  line L31 (20.2722, -36.8985) -> (20.2722, -37.3803)
  line L32 (20.2722, -37.3803) -> (19.8955, -37.4241)
  line L33 (19.8955, -37.4241) -> (19.5187, -37.468)
  line L34 (19.5187, -37.468) -> (19.9655, -37.9761)
  spline S176 degree 3 poles (19.9655, -37.9761) (20.2109, -38.2477) (20.4737, -38.4755) (20.535, -38.4755) knots 0 0 0 0 1 1 1 1
  spline S177 degree 3 poles (20.535, -38.4755) (20.5963, -38.4755) (20.7365, -38.3704) (20.8329, -38.2477) knots 0 0 0 0 1 1 1 1
  line L35 (8.4096, -37.9761) -> (8.8651, -37.468)
  line L36 (8.8651, -37.468) -> (8.4797, -37.4241)
  line L37 (8.4797, -37.4241) -> (8.0942, -37.3803)
  line L38 (8.0942, -37.3803) -> (8.0942, -36.8985)
  spline S178 degree 3 poles (8.0942, -36.8985) (8.0942, -36.6356) (8.1292, -36.2764) (8.1643, -36.11) knots 0 0 0 0 1 1 1 1
  line L39 (8.1643, -36.11) -> (8.2343, -35.8033)
  line L40 (8.2343, -35.8033) -> (8.0591, -36.0224)
  spline S179 degree 3 poles (8.0591, -36.0224) (7.9627, -36.145) (7.7525, -36.4692) (7.6035, -36.7583) knots 0 0 0 0 1 1 1 1
  spline S180 degree 3 poles (7.6035, -36.7583) (7.3757, -37.1876) (7.3319, -37.3365) (7.367, -37.6957) knots 0 0 0 0 1 1 1 1
  spline S181 degree 3 poles (7.367, -37.6957) (7.4108, -38.125) (7.6211, -38.4755) (7.8401, -38.4755) knots 0 0 0 0 1 1 1 1
  spline S182 degree 3 poles (7.8401, -38.4755) (7.8927, -38.4755) (8.1555, -38.2477) (8.4096, -37.9761) knots 0 0 0 0 1 1 1 1
  line L41 (18.6979, -21.6115) -> (19.4763, -20.0548)
  line L42 (19.4763, -20.0548) -> (19.0164, -20.0548)
  spline S183 degree 3 poles (19.0164, -20.0548) (18.5847, -20.0548) (18.5564, -20.0477) (18.5564, -19.8991) knots 0 0 0 0 1 1 1 1
  spline S184 degree 3 poles (18.5564, -19.8991) (18.5564, -19.8071) (18.6838, -18.9226) (18.8394, -17.932) knots 0 0 0 0 1 1 1 1
  spline S185 degree 3 poles (18.8394, -17.932) (19.4409, -14.1533) (19.9716, -10.8134) (20.007, -10.6294) knots 0 0 0 0 1 1 1 1
  line L43 (20.007, -10.6294) -> (20.0353, -10.4313)
  line L44 (20.0353, -10.4313) -> (18.0965, -10.4313)
  spline S186 degree 3 poles (18.0965, -10.4313) (17.028, -10.4313) (16.1505, -10.4172) (16.1505, -10.3959) knots 0 0 0 0 1 1 1 1
  spline S187 degree 3 poles (16.1505, -10.3959) (16.1505, -10.3747) (16.4902, -9.5185) (16.9006, -8.4854) knots 0 0 0 0 1 1 1 1
  spline S188 degree 3 poles (16.9006, -8.4854) (17.3181, -7.4523) (17.6436, -6.589) (17.6224, -6.5749) knots 0 0 0 0 1 1 1 1
  spline S189 degree 3 poles (17.6224, -6.5749) (17.5728, -6.5253) (14.2329, -6.5253) (14.1834, -6.5749) knots 0 0 0 0 1 1 1 1
  spline S190 degree 3 poles (14.1834, -6.5749) (14.1551, -6.6032) (13.9287, -7.1693) (13.6739, -7.8344) knots 0 0 0 0 1 1 1 1
  line L45 (13.6739, -7.8344) -> (13.214, -9.0515)
  line L46 (13.214, -9.0515) -> (12.6408, -9.0727)
  line L47 (12.6408, -9.0727) -> (12.0677, -9.0939)
  line L48 (12.0677, -9.0939) -> (12.0252, -8.5066)
  spline S191 degree 3 poles (12.0252, -8.5066) (11.9969, -8.1811) (11.9757, -7.6787) (11.9757, -7.3886) knots 0 0 0 0 1 1 1 1
  spline S192 degree 3 poles (11.9757, -7.3886) (11.9757, -7.0985) (11.9544, -6.7871) (11.9332, -6.7022) knots 0 0 0 0 1 1 1 1
  line L49 (11.9332, -6.7022) -> (11.8908, -6.5395)
  line L50 (11.8908, -6.5395) -> (10.1925, -6.5395)
  line L51 (10.1925, -6.5395) -> (8.4942, -6.5395)
  line L52 (8.4942, -6.5395) -> (8.5367, -6.9499)
  spline S193 degree 3 poles (8.5367, -6.9499) (8.565, -7.1693) (8.6145, -7.799) (8.6499, -8.3439) knots 0 0 0 0 1 1 1 1
  spline S194 degree 3 poles (8.6499, -8.3439) (8.6853, -8.8887) (8.749, -9.6671) (8.7914, -10.0775) knots 0 0 0 0 1 1 1 1
  spline S195 degree 3 poles (8.7914, -10.0775) (8.8693, -10.8559) (9.3009, -16.0426) (9.4283, -17.7904) knots 0 0 0 0 1 1 1 1
  spline S196 degree 3 poles (9.4283, -17.7904) (9.4707, -18.3565) (9.5203, -18.9014) (9.5415, -19.0146) knots 0 0 0 0 1 1 1 1
  line L53 (9.5415, -19.0146) -> (9.584, -19.2056)
  line L54 (9.584, -19.2056) -> (10.5675, -19.2056)
  spline S197 degree 3 poles (10.5675, -19.2056) (11.1053, -19.2056) (11.5511, -19.2127) (11.5511, -19.2269) knots 0 0 0 0 1 1 1 1
  spline S198 degree 3 poles (11.5511, -19.2269) (11.5511, -19.2339) (11.5016, -19.5099) (11.445, -19.8425) knots 0 0 0 0 1 1 1 1
  spline S199 degree 3 poles (11.445, -19.8425) (11.3176, -20.5501) (11.3105, -21.3143) (11.4167, -21.6752) knots 0 0 0 0 1 1 1 1
  spline S200 degree 3 poles (11.4167, -21.6752) (11.5936, -22.2696) (12.1101, -22.7932) (12.754, -23.0267) knots 0 0 0 0 1 1 1 1
  spline S201 degree 3 poles (12.754, -23.0267) (13.1149, -23.1541) (13.3201, -23.1682) (15.5278, -23.1682) knots 0 0 0 0 1 1 1 1
  line L55 (15.5278, -23.1682) -> (17.9196, -23.1682)
  line L56 (17.9196, -23.1682) -> (18.6979, -21.6115)
  spline S202 degree 3 poles (12.9946, -22.6375) (12.2799, -22.4253) (11.7634, -21.753) (11.7634, -21.0313) knots 0 0 0 0 1 1 1 1
  spline S203 degree 3 poles (11.7634, -21.0313) (11.7634, -20.8261) (11.8271, -20.2741) (11.9049, -19.8071) knots 0 0 0 0 1 1 1 1
  spline S204 degree 3 poles (11.9049, -19.8071) (11.9827, -19.3401) (12.0464, -18.9155) (12.0464, -18.8731) knots 0 0 0 0 1 1 1 1
  spline S205 degree 3 poles (12.0464, -18.8731) (12.0464, -18.8094) (11.7705, -18.7811) (10.9992, -18.7669) knots 0 0 0 0 1 1 1 1
  line L57 (10.9992, -18.7669) -> (9.959, -18.7457)
  line L58 (9.959, -18.7457) -> (9.9095, -18.0381)
  spline S206 degree 3 poles (9.9095, -18.0381) (9.8811, -17.6489) (9.8104, -16.7573) (9.7467, -16.0568) knots 0 0 0 0 1 1 1 1
  spline S207 degree 3 poles (9.7467, -16.0568) (9.5627, -13.941) (9.4424, -12.448) (9.3221, -10.9974) knots 0 0 0 0 1 1 1 1
  spline S208 degree 3 poles (9.3221, -10.9974) (9.2585, -10.2403) (9.1806, -9.2708) (9.1452, -8.8392) knots 0 0 0 0 1 1 1 1
  spline S209 degree 3 poles (9.1452, -8.8392) (9.1099, -8.4146) (9.0603, -7.8132) (9.032, -7.5089) knots 0 0 0 0 1 1 1 1
  line L59 (9.032, -7.5089) -> (8.9896, -6.964)
  line L60 (8.9896, -6.964) -> (10.2279, -6.964)
  line L61 (10.2279, -6.964) -> (11.4733, -6.964)
  line L62 (11.4733, -6.964) -> (11.5086, -7.332)
  spline S210 degree 3 poles (11.5086, -7.332) (11.5299, -7.5372) (11.5653, -8.1104) (11.5936, -8.6057) knots 0 0 0 0 1 1 1 1
  line L63 (11.5936, -8.6057) -> (11.636, -9.5114)
  line L64 (11.636, -9.5114) -> (12.5771, -9.5114)
  line L65 (12.5771, -9.5114) -> (13.5112, -9.5114)
  line L66 (13.5112, -9.5114) -> (13.9923, -8.2377)
  line L67 (13.9923, -8.2377) -> (14.4735, -6.964)
  line L68 (14.4735, -6.964) -> (15.7331, -6.964)
  spline S211 degree 3 poles (15.7331, -6.964) (16.4336, -6.964) (16.9997, -6.9782) (16.9997, -6.9994) knots 0 0 0 0 1 1 1 1
  spline S212 degree 3 poles (16.9997, -6.9994) (16.9997, -7.0277) (15.6198, -10.4809) (15.4642, -10.8417) knots 0 0 0 0 1 1 1 1
  spline S213 degree 3 poles (15.4642, -10.8417) (15.4359, -10.9054) (15.8604, -10.9266) (17.4525, -10.9266) knots 0 0 0 0 1 1 1 1
  spline S214 degree 3 poles (17.4525, -10.9266) (19.7452, -10.9266) (19.5329, -10.8559) (19.4055, -11.5706) knots 0 0 0 0 1 1 1 1
  spline S215 degree 3 poles (19.4055, -11.5706) (19.3702, -11.7828) (19.2711, -12.3843) (19.1933, -12.9079) knots 0 0 0 0 1 1 1 1
  spline S216 degree 3 poles (19.1933, -12.9079) (19.1083, -13.4316) (18.9668, -14.3444) (18.8748, -14.9246) knots 0 0 0 0 1 1 1 1
  spline S217 degree 3 poles (18.8748, -14.9246) (18.7828, -15.5119) (18.6342, -16.4177) (18.5564, -16.9413) knots 0 0 0 0 1 1 1 1
  spline S218 degree 3 poles (18.5564, -16.9413) (18.4715, -17.4649) (18.3441, -18.2858) (18.2663, -18.7528) knots 0 0 0 0 1 1 1 1
  spline S219 degree 3 poles (18.2663, -18.7528) (18.1955, -19.2269) (18.1106, -19.8071) (18.0894, -20.0477) knots 0 0 0 0 1 1 1 1
  line L69 (18.0894, -20.0477) -> (18.0399, -20.4793)
  line L70 (18.0399, -20.4793) -> (18.3724, -20.4793)
  spline S220 degree 3 poles (18.3724, -20.4793) (18.5493, -20.4793) (18.6979, -20.5147) (18.6979, -20.5501) knots 0 0 0 0 1 1 1 1
  spline S221 degree 3 poles (18.6979, -20.5501) (18.6979, -20.5926) (18.4573, -21.102) (18.1672, -21.6823) knots 0 0 0 0 1 1 1 1
  line L71 (18.1672, -21.6823) -> (17.6365, -22.7437)
  line L72 (17.6365, -22.7437) -> (15.4925, -22.7437)
  spline S222 degree 3 poles (15.4925, -22.7437) (13.8084, -22.7437) (13.2706, -22.7224) (12.9946, -22.6375) knots 0 0 0 0 1 1 1 1
  spline S223 degree 3 poles (17.7285, -21.6469) (17.9125, -21.2789) (18.0611, -20.9605) (18.0611, -20.9393) knots 0 0 0 0 1 1 1 1
  spline S224 degree 3 poles (18.0611, -20.9393) (18.0611, -20.9181) (17.9479, -20.9039) (17.8063, -20.9039) knots 0 0 0 0 1 1 1 1
  line L73 (17.8063, -20.9039) -> (17.5445, -20.9039)
  line L74 (17.5445, -20.9039) -> (17.587, -20.5713)
  spline S225 degree 3 poles (17.587, -20.5713) (17.6153, -20.3803) (17.7144, -19.7363) (17.8134, -19.1349) knots 0 0 0 0 1 1 1 1
  spline S226 degree 3 poles (17.8134, -19.1349) (17.9125, -18.5334) (18.054, -17.6277) (18.1318, -17.1182) knots 0 0 0 0 1 1 1 1
  spline S227 degree 3 poles (18.1318, -17.1182) (18.2097, -16.6158) (18.3158, -15.9153) (18.3724, -15.5615) knots 0 0 0 0 1 1 1 1
  spline S228 degree 3 poles (18.3724, -15.5615) (18.429, -15.2147) (18.5918, -14.1958) (18.7262, -13.2971) knots 0 0 0 0 1 1 1 1
  spline S229 degree 3 poles (18.7262, -13.2971) (18.8678, -12.4055) (18.9951, -11.5847) (19.0164, -11.4786) knots 0 0 0 0 1 1 1 1
  line L75 (19.0164, -11.4786) -> (19.0447, -11.2804)
  line L76 (19.0447, -11.2804) -> (17.0846, -11.2804)
  line L77 (17.0846, -11.2804) -> (15.1174, -11.2804)
  line L78 (15.1174, -11.2804) -> (14.0773, -13.8844)
  spline S230 degree 3 poles (14.0773, -13.8844) (13.5112, -15.3138) (13.0229, -16.538) (12.9946, -16.6087) knots 0 0 0 0 1 1 1 1
  spline S231 degree 3 poles (12.9946, -16.6087) (12.9592, -16.7078) (12.9946, -16.729) (13.1715, -16.729) knots 0 0 0 0 1 1 1 1
  spline S232 degree 3 poles (13.1715, -16.729) (13.2918, -16.729) (13.3909, -16.7432) (13.3909, -16.7644) knots 0 0 0 0 1 1 1 1
  spline S233 degree 3 poles (13.3909, -16.7644) (13.3909, -16.7856) (13.1857, -17.2102) (12.938, -17.7055) knots 0 0 0 0 1 1 1 1
  spline S234 degree 3 poles (12.938, -17.7055) (12.5205, -18.5476) (12.4781, -18.6679) (12.3365, -19.5453) knots 0 0 0 0 1 1 1 1
  spline S235 degree 3 poles (12.3365, -19.5453) (12.096, -21.0666) (12.1384, -21.562) (12.5559, -21.937) knots 0 0 0 0 1 1 1 1
  spline S236 degree 3 poles (12.5559, -21.937) (12.9592, -22.312) (13.0229, -22.3191) (15.2802, -22.3191) knots 0 0 0 0 1 1 1 1
  line L79 (15.2802, -22.3191) -> (17.3889, -22.3191)
  line L80 (17.3889, -22.3191) -> (17.7285, -21.6469)
  spline S237 degree 3 poles (13.957, -20.7978) (13.8791, -20.7058) (13.9145, -20.352) (14.1622, -18.7952) knots 0 0 0 0 1 1 1 1
  spline S238 degree 3 poles (14.1622, -18.7952) (14.5655, -16.3045) (14.9264, -14.0543) (15.0254, -13.4386) knots 0 0 0 0 1 1 1 1
  spline S239 degree 3 poles (15.0254, -13.4386) (15.0679, -13.1698) (15.1387, -12.9009) (15.174, -12.8584) knots 0 0 0 0 1 1 1 1
  spline S240 degree 3 poles (15.174, -12.8584) (15.2307, -12.7947) (15.5137, -12.7664) (16.1718, -12.7664) knots 0 0 0 0 1 1 1 1
  line L81 (16.1718, -12.7664) -> (17.0917, -12.7664)
  line L82 (17.0917, -12.7664) -> (17.0421, -13.1415)
  spline S241 degree 3 poles (17.0421, -13.1415) (16.9926, -13.5165) (16.7732, -14.9317) (16.3204, -17.7551) knots 0 0 0 0 1 1 1 1
  spline S242 degree 3 poles (16.3204, -17.7551) (16.1859, -18.6113) (16.0232, -19.6302) (15.9666, -20.0194) knots 0 0 0 0 1 1 1 1
  spline S243 degree 3 poles (15.9666, -20.0194) (15.9029, -20.4086) (15.8463, -20.7695) (15.8321, -20.819) knots 0 0 0 0 1 1 1 1
  spline S244 degree 3 poles (15.8321, -20.819) (15.7826, -20.9605) (14.0773, -20.9393) (13.957, -20.7978) knots 0 0 0 0 1 1 1 1
  spline S245 degree 3 poles (12.7045, -17.6843) (12.8885, -17.3163) (13.0371, -16.9979) (13.0371, -16.9767) knots 0 0 0 0 1 1 1 1
  spline S246 degree 3 poles (13.0371, -16.9767) (13.0371, -16.9555) (12.9592, -16.9413) (12.8602, -16.9413) knots 0 0 0 0 1 1 1 1
  spline S247 degree 3 poles (12.8602, -16.9413) (12.7611, -16.9413) (12.6833, -16.913) (12.6833, -16.8705) knots 0 0 0 0 1 1 1 1
  spline S248 degree 3 poles (12.6833, -16.8705) (12.6833, -16.8352) (13.5041, -14.7406) (14.516, -12.2216) knots 0 0 0 0 1 1 1 1
  spline S249 degree 3 poles (14.516, -12.2216) (15.5208, -9.6954) (16.3699, -7.5655) (16.3911, -7.4806) knots 0 0 0 0 1 1 1 1
  spline S250 degree 3 poles (16.3911, -7.4806) (16.4407, -7.3178) (16.4407, -7.3178) (15.5845, -7.3178) knots 0 0 0 0 1 1 1 1
  spline S251 degree 3 poles (15.5845, -7.3178) (14.9618, -7.3178) (14.7212, -7.3391) (14.6999, -7.4098) knots 0 0 0 0 1 1 1 1
  spline S252 degree 3 poles (14.6999, -7.4098) (14.6858, -7.4523) (14.4806, -8.0255) (14.2329, -8.6835) knots 0 0 0 0 1 1 1 1
  line L83 (14.2329, -8.6835) -> (13.7942, -9.8652)
  line L84 (13.7942, -9.8652) -> (12.5417, -9.8652)
  line L85 (12.5417, -9.8652) -> (11.2822, -9.8652)
  line L86 (11.2822, -9.8652) -> (11.2398, -9.0727)
  spline S253 degree 3 poles (11.2398, -9.0727) (11.2114, -8.634) (11.1761, -8.0608) (11.1548, -7.799) knots 0 0 0 0 1 1 1 1
  line L87 (11.1548, -7.799) -> (11.1124, -7.3178)
  line L88 (11.1124, -7.3178) -> (10.2703, -7.3178)